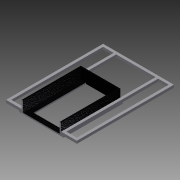
# Autodesk Inventor part: Robot frame
Saved by Autodesk Inventor 2014 SP1 (Build 180222100, 222)
## iProperties
Created: 2014-01-07
Part Number: Robot frame
Material: Generic
Document SubType Name: Modeling
Designer: ju brian
Density: 1 g/cm^3
Appearance: Default
Author: ju brian
Autodesk Inventor part; units mm, degrees
ref_plane "YZ Plane" through (0, 0, 0) normal (1, 0, 0) x (0, 1, 0)
ref_plane "XZ Plane" through (0, 0, 0) normal (0, 1, 0) x (-1, 0, 0)
sketch "Sketch1" plane through (0, 0, 0) normal (0, 1, 0) x (-1, 0, 0)
  line L0 (-6.5808, 12.0286) -> (-6.5808, -927.7714)
  line L1 (-6.5808, 12.0286) -> (18.8192, 12.0286)
  line L2 (18.8192, 12.0286) -> (18.8192, -902.3714)
  line L3 (18.8192, -902.3714) -> (653.8192, -902.3714)
  line L4 (653.8192, -902.3714) -> (653.8192, 12.0286)
  line L5 (653.8192, 12.0286) -> (679.2192, 12.0286)
  line L6 (679.2192, 12.0286) -> (679.2192, -927.7714)
  line L7 (679.2192, -927.7714) -> (-6.5808, -927.7714)
  line L8 (18.8192, 12.0286) -> (145.8192, 12.0286)
  line L9 (145.8192, 12.0286) -> (145.8192, -902.3714)
  line L10 (145.8192, -902.3714) -> (120.4192, -902.3714)
  line L11 (120.4192, -902.3714) -> (120.4192, 12.0286)
  line L12 (120.4192, -13.8644) -> (18.8192, -13.8644)
  line L13 (653.8192, 12.0286) -> (526.8192, 12.0286)
  line L14 (526.8192, 12.0286) -> (526.8192, -902.3714)
  line L15 (552.2192, 12.0286) -> (552.2192, -902.3714)
  line L16 (552.2192, -13.8644) -> (653.8192, -13.8644)
  point P0 (69.6192, -13.8644)
  dimension "d0" = 939.8
  dimension "d1" = 25.4
  dimension "d2" = 914.4
  dimension "d3" = 635
  dimension "d5" = 25.4
  dimension "d6" = 90
  dimension "d9" = 127
  dimension "d11" = 25.4
  dimension "d12" = 127
  dimension "d21" = 25.4
  constraints: 34 end point, 11 point on line, 8 perpendicular, 4 parallel, 2 collinear, 1 midpoint, 1 vertical
  measures "d0" distance of L0.start L0.end
  measures "d1" distance of L0.start L1.end
  measures "d2" distance of L1.end L2.end
  measures "d3" distance of L2.end L3.end
  measures "d5" distance of L4.end L5.end
  measures "d6" angle of L4 L5
  measures "d9" distance of L1.end L8.end
  measures "d11" distance of L9.end L10.end
  measures "d12" distance of L4.end L13.end
  measures "d21" distance between parallel lines of L14 L15
extrude "Extrusion1" add sketch "Sketch1" along normal mid plane 25.4 contours L1 L2 L3 L4 L5 L6 L7 L0 | L8 L11 L12 L2 | L8 L9 L3 L11 | L4 L16 L15 L13 | L15 L3 L14 L13
sketch "Sketch2" plane through (-526.8192, -12.7, -902.3714) normal (1, 0, 0) x (0, 0, -1)
  line L0 (-914.4, 0) -> (-355.6, 0)
  line L1 (-355.6, 0) -> (-355.6, 101.6)
  line L2 (-355.6, 101.6) -> (-914.4, 101.6)
  line L3 (-914.4, 101.6) -> (-914.4, 0)
  dimension "d14" = 558.8
  dimension "d16" = 101.6
  constraints: 8 end point, 2 parallel, 1 horizontal, 1 perpendicular
  measures "d14" distance of L1.end L2.end
  measures "d16" distance of L2.end L0.start
extrude "Extrusion2" add sketch "Sketch2" along normal blind 12.7
ref_plane "Work Plane1" through (-336.3192, 12.7, -902.3714) normal (1, 0, 0) x (0, -1, 0)
mirror "Mirror1" about plane through (-336.3192, 12.7, -902.3714) normal (1, 0, 0) of "Extrusion2"
sketch "Sketch3" plane through (-145.8192, 12.7, -546.7714) normal (0, 0, -1) x (-1, 0, 0)
  line L0 (0, 76.2) -> (381, 76.2)
  line L1 (381, 76.2) -> (381, -25.4)
  line L2 (381, -25.4) -> (0, -25.4)
  line L3 (0, -25.4) -> (0, 76.2)
  constraints: 8 end point, 2 parallel, 1 horizontal, 1 perpendicular
extrude "Extrusion3" add sketch "Sketch3" along normal blind 12.7
sketch "Sketch4" plane through (0, -12.7, 0) normal (0, -1, 0) x (1, 0, 0)
  line L0 (6.5808, 12.0286) -> (-158.5192, 12.0286) projected
  line L1 (-552.2192, -902.3714) -> (-552.2192, -13.8644) projected
  line L2 (-552.2192, -559.4714) -> (-120.4192, -559.4714)
  line L3 (-120.4192, -559.4714) -> (-120.4192, 12.0286)
  line L4 (-120.4192, 12.0286) -> (-552.2192, 12.0286)
  line L5 (-552.2192, 12.0286) -> (-552.2192, -559.4714)
  constraints: 8 end point, 2 parallel, 2 point on line, 1 horizontal, 1 perpendicular
extrude "Extrusion4" add sketch "Sketch4" along normal blind 12.7
sketch "Sketch5" plane through (0, -12.7, 0) normal (0, 1, 0) x (1, 0, 0)
  line L0 (-514.1192, -12.0286) -> (-514.1192, 546.7714) projected
  line L1 (-158.5192, 546.7714) -> (-514.1192, 546.7714) projected
  line L2 (-463.3192, 546.7714) -> (-209.3192, 546.7714)
  line L3 (-209.3192, 546.7714) -> (-209.3192, 38.7714)
  line L4 (-209.3192, 38.7714) -> (-463.3192, 38.7714)
  line L5 (-463.3192, 38.7714) -> (-463.3192, 546.7714)
  point P0 (-336.3192, 38.7714)
  dimension "d24" = 254
  dimension "d25" = 508
  dimension "d26" = 177.8
  constraints: 8 end point, 2 parallel, 1 horizontal, 1 midpoint, 1 perpendicular, 1 point on line
  measures "d24" distance of L3.end L4.end
  measures "d25" distance of L2.end L3.end
  measures "d26" distance from line of L0 point (-336.319, 38.771)
extrude "Extrusion5" cut sketch "Sketch5" against normal blind 12.7
body "Solid1"
